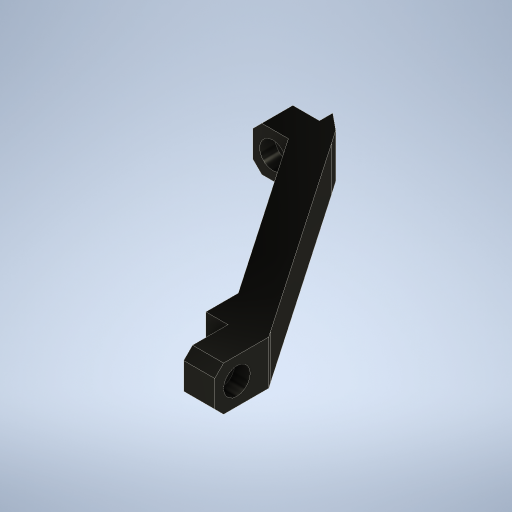
# Autodesk Inventor part: HoldingArms
Saved by Autodesk Inventor 2024.3 (Build 283343000, 343)
## iProperties
Created: 2025-01-30
Part Number: HoldingArms
Material: Generic
Document SubType Name: Modeling
Designer: migue
Density: 1 g/cm^3
Appearance: Gunmetal
Author: migue
Autodesk Inventor part; units mm, degrees
ref_plane "YZ Plane" through (0, 0, 0) normal (1, 0, 0) x (0, 1, 0)
ref_plane "XZ Plane" through (0, 0, 0) normal (0, 1, 0) x (-1, 0, 0)
ref_plane "XY Plane" through (0, 0, 0) normal (0, 0, 1) x (1, 0, 0)
sketch "Sketch1" plane through (0, 0, 0) normal (0, 1, 0) x (-1, 0, 0)
  line L0 (0, 0) -> (7, 0)
  line L1 (7, 0) -> (7, -10)
  line L2 (7, -10) -> (0, -10)
  line L3 (0, -10) -> (0, 0)
  line L4 (36.5, -60.1) -> (44.5, -60.1)
  line L5 (44.5, -60.1) -> (44.5, -53.1)
  line L6 (44.5, -53.1) -> (36.5, -53.1)
  line L7 (36.5, -53.1) -> (36.5, -60.1)
  line L8 (36.5, -53.1) -> (7, -10)
  line L9 (30.7235, -57.0537) -> (0.8012, -13.3368)
  line L10 (0.8012, -13.3368) -> (0, -12.1913)
  line L11 (0, -12.1913) -> (0, -10)
  line L12 (30.7235, -57.0537) -> (32.8378, -60.1)
  line L13 (32.8378, -60.1) -> (36.5, -60.1)
  dimension "d0" = 10
  dimension "d1" = 7
  dimension "d7" = 29.5
  dimension "d14" = 50.1
  dimension "d15" = 7
  dimension "d16" = 8
  dimension "d17" = 7
  constraints: 28 end point, 5 parallel, 3 perpendicular, 2 horizontal, 1 vertical
  measures "d0" distance of L2.end L0.start
  measures "d1" distance of L0.start L0.end
  measures "d7" distance from line of L1 L4.start
  measures "d14" distance from line of L2 L4.start
  measures "d15" distance of L4.end L5.end
  measures "d16" distance of L4.start L4.end
  measures "d17" distance between parallel lines of L8 L9
extrude "Extrusion1" add sketch "Sketch1" along normal blind 10
chamfer "Chamfer1" distance 2 angle 45 4 edges at (-44.5, 0, -56.6) (-44.5, 10, -56.6) (-3.5, 10, 0) (-3.5, 0, 0)
sketch "Sketch2" plane through (0, 0, -12.1913) normal (1, 0, 0) x (0, 0, -1)
  line L0 (-12.1913, 0) -> (-2.1913, 0) construction
  line L1 (-2.1913, 0) -> (-2.1913, 10) construction
  line L2 (-2.1913, 10) -> (-12.1913, 10) construction
  line L3 (-12.1913, 10) -> (-12.1913, 0) construction
  line L4 (-2.1913, 10) -> (-12.1913, 0) construction
  circle A0 centre (-7.1913, 5) radius 1.6
  dimension "d21" = 10
  dimension "d22" = 10
  dimension "d23" = 3.2
  constraints: 10 end point, 2 parallel, 1 centre point, 1 horizontal, 1 midpoint, 1 perpendicular
  measures "d21" distance of L2.end L1.end
  measures "d22" distance of L1.end L0.end
  measures "d23" diameter of A0
extrude "Extrusion2" cut sketch "Sketch2" against normal through all
sketch "Sketch3" plane through (-36.5, 0, -53.1) normal (0, 0, 1) x (1, 0, 0)
  line L0 (0, 0) -> (0, 10) projected
  line L1 (0, 10) -> (-10, 0) construction
  line L2 (0, 10) -> (14.1421, 10) construction
  line L3 (0, 5) -> (-3.5, 5)
  circle A0 centre (-3.5, 5) radius 1.5
  point P0 (36.5, 0)
  dimension "d26" = 135
  dimension "d27" = 3.5
  dimension "d28" = 3
  constraints: 6 end point, 2 horizontal, 1 centre point, 1 coincident, 1 equal length, 1 midpoint
  measures "d26" angle of L1 L2
  measures "d27" distance of L3.start L3.end
  measures "d28" diameter of A0
extrude "Extrusion3" cut sketch "Sketch3" against normal blind 10
sketch "Sketch4" plane through (0, 0, -12.1913) normal (1, 0, 0) x (0, 0, -1)
  circle A0 centre (-7.1913, 5) radius 1.6 projected
  circle A1 centre (-7.1913, 5) radius 3
  point P0 (-12.1913, 0)
  dimension "d31" = 6
  constraints: 1 centre point, 1 coincident
  measures "d31" diameter of A1
extrude "Extrusion4" cut sketch "Sketch4" against normal blind 3.5
sketch "Sketch5" plane through (-36.5, 0, -53.1) normal (0, 0, 1) x (1, 0, 0)
  circle A0 centre (-3.5, 5) radius 3
  point P0 (36.5, 0)
  dimension "d34" = 6
  constraints: 1 centre point
  measures "d34" diameter of A0
extrude "Extrusion5" cut sketch "Sketch5" against normal blind 3.5
sketch "Sketch6" plane through (0, 10, 0) normal (0, 1, 0) x (1, 0, 0)
  line L0 (-7, 10) -> (-7, 2) projected
  line L1 (-7, 10) -> (-12, 10)
  line L2 (-12, 10) -> (-12, 17.3051)
  line L3 (-36.5, 53.1) -> (-7, 10) projected
  point P0 (0, 0)
  dimension "d37" = 5
  dimension "d38" = 90
  constraints: 4 end point, 1 horizontal, 1 point on line
  measures "d37" distance of L0.start L1.end
  measures "d38" angle of L1 L2
extrude "Extrusion6" add sketch "Sketch6" against normal blind 10
sketch "Sketch7" plane through (0, 10, 0) normal (0, 1, 0) x (1, 0, 0)
  line L0 (-30.7235, 57.0537) -> (-32.8378, 60.1) projected
  line L1 (-32.8378, 60.1) -> (-36.4998, 60.1)
  line L2 (-32.8378, 60.1) -> (-42.5, 60.1) projected
  line L3 (-36.4998, 60.1) -> (-36.4998, 63.1)
  line L4 (-36.4998, 63.1) -> (-32.8378, 60.1)
  point P0 (0, 0)
  dimension "d41" = 3.662
  dimension "d42" = 3
  constraints: 6 end point, 1 point on line, 1 vertical
  measures "d41" distance of L0.end L1.end
  measures "d42" distance of L1.end L3.end
extrude "Extrusion7" add sketch "Sketch7" against normal blind 10
body "Solid1"
